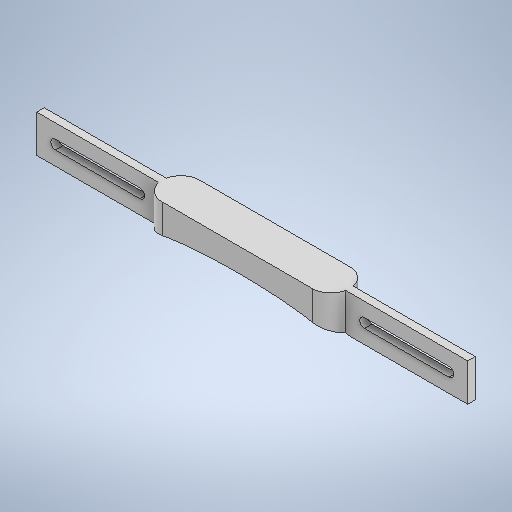
# Autodesk Inventor part: AllFretBars
Saved by Autodesk Inventor 2025.1 (Build 291241000, 241)
## iProperties
Created: 2025-11-05
Part Number: AllFretBars
Material: Generic
Document SubType Name: Modeling
Designer: Juxin
Density: 1 g/cm^3
Appearance: Default
Author: Juxin
Autodesk Inventor part; units mm, degrees
ref_plane "YZ Plane" through (0, 0, 0) normal (1, 0, 0) x (0, 1, 0)
ref_plane "XZ Plane" through (0, 0, 0) normal (0, 1, 0) x (-1, 0, 0)
ref_plane "XY Plane" through (0, 0, 0) normal (0, 0, 1) x (1, 0, 0)
sketch "Sketch1" plane through (0, 0, 0) normal (0, 1, 0) x (-1, 0, 0)
  line L0 (-17.4625, -7.85) -> (-17.4625, -5.31)
  line L1 (-17.4625, -6.35) -> (-17.4625, -5.31)
  line L2 (-17.4625, -5.31) -> (-1.5875, -5.31)
  line L3 (-1.5875, -7.85) -> (-17.4625, -7.85)
  line L4 (-1.5875, -5.31) -> (-1.5875, -0.23)
  line L5 (-1.5875, -7.85) -> (-1.5875, -12.93)
  line L6 (-1.5875, -0.23) -> (30, -0.23)
  line L7 (-1.5875, -12.93) -> (30, -12.93)
  line L8 (30, -12.93) -> (30, -0.23)
  line L9 (61.5875, -7.85) -> (77.4625, -7.85)
  line L10 (77.4625, -5.31) -> (61.5875, -5.31)
  line L11 (77.4625, -7.85) -> (77.4625, -5.31)
  line L12 (77.4625, -6.35) -> (77.4625, -5.31)
  line L13 (61.5875, -7.85) -> (61.5875, -12.93)
  line L14 (61.5875, -5.31) -> (61.5875, -0.23)
  line L15 (61.5875, -0.23) -> (30, -0.23)
  line L16 (61.5875, -12.93) -> (30, -12.93)
  point P0 (-17.4625, -6.58)
  point P1 (77.4625, -6.58)
  dimension "d135" = 6.35
  dimension "d136" = 2.54
  constraints: 34 end point, 8 symmetric about line, 4 point on line, 1 midpoint, 1 vertical
  measures "d135" vertical distance of L4.end point (-17.462, -6.58)
  measures "d136" distance of L3.end L2.start
extrude "Extrusion1" add sketch "Sketch1" along normal blind 12.7
fillet "Fillet2" radius 6.35 4 edges at (1.5875, 6.35, -12.93) (1.5875, 6.35, -0.23) (-61.5875, 6.35, -12.93) (-61.5875, 6.35, -0.23)
move faces "Move4" translate (25.4, 0, 0) faces at (17.4625, 4.2333, -6.1567)
move faces "Move5" translate (-25.4, 0, 0) faces at (-77.4625, 4.2333, -7.0033)
sketch "Sketch6" plane through (-55.3658, 0, -0.23) normal (0, 0, 1) x (1, 0, 0)
  line L0 (50.7316, 0) -> (0, 0) projected
  line L1 (56.9533, 0) -> (50.7316, 0) projected
  ellipse E0 centre (25.3658, 0) end of major axis (56.9533, 0) minor radius 4.7022
  point P0 (55.3658, 0)
  constraints: 1 horizontal, 1 horizontal alignment, 1 midpoint, 2 other
extrude "Extrusion18" cut sketch "Sketch6" against normal blind 20.6375
fillet "Fillet4" radius 3.175 2 edges at (-61.5875, 0, -6.58) (1.5875, 0, -6.58)
sketch "Sketch7" plane through (-102.8625, 12.7, -5.31) normal (0, 0, 1) x (1, 0, 0)
  line L0 (41.275, -12.2395) -> (41.275, 0) projected
  line L1 (41.275, -6.1198) -> (50.8, -6.1198) construction
  line L2 (0, -12.7) -> (0, 0) projected
  line L3 (0, -6.35) -> (6.35, -6.35)
  line L4 (0, -6.35) -> (6.35, -6.35) construction
  line L5 (41.275, -6.35) -> (34.925, -6.35)
  line L6 (41.275, -6.35) -> (47.625, -6.35) construction
  arc A0 (34.925, -7.9375) -> (34.925, -4.7625) centre (34.925, -6.35) ccw
  arc A1 (6.35, -4.7625) -> (6.35, -7.9375) centre (6.35, -6.35) ccw
  line L7 (6.35, -4.7625) -> (34.925, -4.7625)
  line L8 (34.925, -7.9375) -> (6.35, -7.9375)
  line L9 (98.2283, 0) -> (47.4967, 0) projected
  line L10 (72.8625, 0) -> (72.8625, -18.9978)
  line L11 (145.725, -6.35) -> (139.375, -6.35)
  line L12 (104.45, -6.35) -> (110.8, -6.35)
  arc A2 (110.8, -4.7625) -> (110.8, -7.9375) centre (110.8, -6.35) ccw
  arc A3 (139.375, -7.9375) -> (139.375, -4.7625) centre (139.375, -6.35) ccw
  line L13 (139.375, -4.7625) -> (110.8, -4.7625)
  line L14 (110.8, -7.9375) -> (139.375, -7.9375)
  point P0 (102.8625, -12.7)
  dimension "d152" = 6.35
  dimension "d153" = 0
  dimension "d154" = 6.35
  dimension "d155" = 180
  dimension "d156" = 3.175
  dimension "d157" = 3.175
  constraints: 24 end point, 10 symmetric about line, 8 point on circle, 5 horizontal, 4 centre point, 3 coincident, 3 midpoint, 2 collinear, 2 tangent, 1 point on line, 1 vertical, 2 other
  measures "d152" distance of L3.start L3.end
  measures "d153" distance between parallel lines of L3 L4
  measures "d154" distance of L5.start L5.end
  measures "d155" angle of L5 L6
  measures "d156" diameter of A0
  measures "d157" diameter of A1
extrude "Extrusion19" cut sketch "Sketch7" against normal blind 20.6375
body "Solid1"
